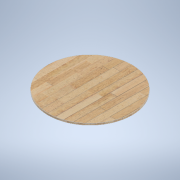
# Autodesk Inventor part: Plateau
Saved by Autodesk Inventor 2021 (Build 250183000, 183)
## iProperties
Created: 2021-01-25
Part Number: Plateau
Material: Bois (Erable)
Document SubType Name: Modeling
Designer: dimercur
Density: 0.67 g/cm^3
Appearance: Erable naturel - Lustré teinte foncée
Author: dimercur
Autodesk Inventor part; units mm, degrees
ref_plane "YZ Plane" through (0, 0, 0) normal (1, 0, 0) x (0, 1, 0)
ref_plane "XZ Plane" through (0, 0, 0) normal (0, 1, 0) x (-1, 0, 0)
ref_plane "XY Plane" through (0, 0, 0) normal (0, 0, 1) x (1, 0, 0)
sketch "Esquisse1" plane through (0, 0, 0) normal (0, 1, 0) x (-1, 0, 0)
  circle A0 centre (0, 0) radius 350
  dimension "d0" = 700
  constraints: 1 centre point, 1 coincident
  measures "d0" diameter of A0
extrude "Extrusion1" add sketch "Esquisse1" along normal blind 15
sketch "Esquisse2" plane through (0, 15, 0) normal (0, 1, 0) x (1, 0, 0)
  circle A0 centre (260, -59.5) radius 1.25
  circle A1 centre (200, -59.5) radius 1.25
  circle A2 centre (200, 59.5) radius 1.25
  circle A3 centre (260, 59.5) radius 1.25
  point P0 (0, 0)
  dimension "d3" = 2.5
  dimension "d4" = 2.5
  dimension "d5" = 2.5
  dimension "d6" = 2.5
  dimension "d7" = 119
  dimension "d8" = 119
  dimension "d9" = 60
  dimension "d10" = 59.5
  dimension "d11" = 200
  constraints: 4 centre point
  measures "d3" diameter of A1
  measures "d4" diameter of A0
  measures "d5" diameter of A2
  measures "d6" diameter of A3
  measures "d7" distance of A2.centre A1.centre
  measures "d8" distance of A3.centre A0.centre
  measures "d9" distance of A0.centre A1.centre
  measures "d10" vertical distance of point (0, 0) A1.centre
  measures "d11" horizontal distance of point (0, 0) A1.centre
extrude "Extrusion2" cut sketch "Esquisse2" against normal blind 10
equation "\"d4\" = d3"
equation "\"d5\" = d3"
equation "\"d6\" = d3"
equation "\"d8\" = d7"
equation "\"d10\" = 0.5 * d7"
